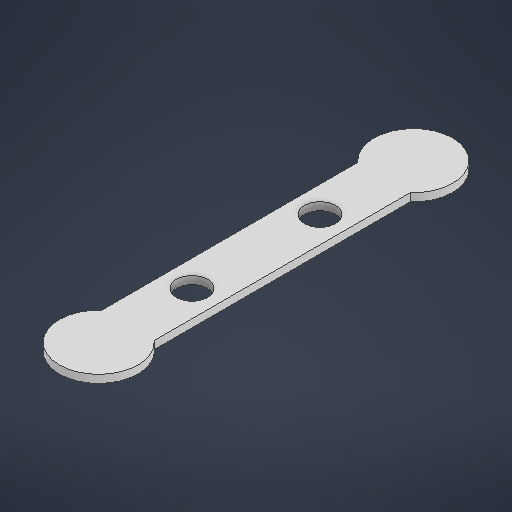
# Autodesk Inventor part: ramenovaPricka
Saved by Autodesk Inventor 2026 (Build 300175000, 175)
## iProperties
Created: 2025-04-11
Part Number: ramenovaPricka
Material: Generic
Document SubType Name: Modeling
Designer: vitgr
Density: 1 g/cm^3
Appearance: Default
Author: vitgr
Autodesk Inventor part; units mm, degrees
ref_plane "YZ Plane" through (0, 0, 0) normal (1, 0, 0) x (0, 1, 0)
ref_plane "XZ Plane" through (0, 0, 0) normal (0, 1, 0) x (-1, 0, 0)
ref_plane "XY Plane" through (0, 0, 0) normal (0, 0, 1) x (1, 0, 0)
sketch "Sketch1" plane through (0, 0, 0) normal (0, 1, 0) x (-1, 0, 0)
  line L0 (0, 0) -> (0, 75)
  line L1 (0, 0) -> (0, -75)
  line L2 (0, -75) -> (0, -60)
  circle A0 centre (0, -60) radius 15
  circle A1 centre (0, 60) radius 15
  line L3 (-10, 45) -> (-10, -48.8197)
  line L4 (10, 45) -> (10, -48.8197)
  line L5 (10, 45) -> (10, 48.8197)
  line L6 (-10, 45) -> (-10, 48.8197)
  line L7 (10, 45) -> (-10, 45)
  line L8 (-10, -48.8197) -> (-10, 0)
  line L9 (0, -24.4098) -> (10, -24.4098)
  line L10 (10, 0) -> (0, 0)
  line L11 (0, 24.4098) -> (10, 24.4098)
  line L12 (0, -24.4098) -> (-10, -24.4098)
  line L13 (0, 24.4098) -> (-10, 24.4098)
  circle A2 centre (0, -24.4098) radius 6
  circle A3 centre (0, 24.4098) radius 6
  dimension "d1" = 75
  dimension "d2" = 75
  dimension "d3" = 15
  dimension "d6" = 20
  dimension "d7" = 97.6393
  dimension "d10" = 12
  dimension "d11" = 12
  constraints: 28 end point, 5 point on circle, 4 centre point, 4 point on line, 4 symmetric about line, 3 coincident, 3 vertical, 2 perpendicular, 1 horizontal, 1 parallel
  measures "d1" distance of L0.start L0.end
  measures "d2" distance of L0.start L1.end
  measures "d3" distance of L1.end L2.end
  measures "d6" distance of L4.start L3.start
  measures "d7" distance of L3.end L6.end
  measures "d10" diameter of A2
  measures "d11" diameter of A3
extrude "Extrusion1" add sketch "Sketch1" along normal blind 3 contours L1 A2 L12 L3 L13 A3 L0 | L10 L4 L9 A2 L1 | L0 A3 L11 L4 L10 | L13 L3 L7 L0 A3 | A3 L0 L7 L4 L11 | L9 L4 A0 L1 A2 | A2 L1 A0 L3 L12 | L7 A1 L5 | A0 L1 | A1 L0 | L7 L6 A1 | L0 A1 | L1 A0
body "Solid1"
